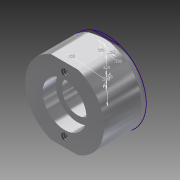
# Autodesk Inventor part: Pnuematic Connector
Saved by Autodesk Inventor 2013 (Build 170138000, 138)
## iProperties
Created: 2013-06-07
Part Number: Pnuematic Connector
Material: Generic
Document SubType Name: Modeling
Designer: mvarma
Density: 1 g/cm^3
Author: mvarma
Autodesk Inventor part; units mm, degrees
ref_plane "YZ Plane" through (0, 0, 0) normal (1, 0, 0) x (0, 1, 0)
ref_plane "XZ Plane" through (0, 0, 0) normal (0, 1, 0) x (-1, 0, 0)
ref_plane "XY Plane" through (0, 0, 0) normal (0, 0, 1) x (1, 0, 0)
sketch "Sketch1" plane through (0, 0, 0) normal (0, 0, 1) x (1, 0, 0)
  circle A0 centre (0, 0) radius 3.175
  line L0 (-1.508, 2.794) -> (1.508, 2.794)
  line L1 (-3.175, 0) -> (0, 0)
  line L2 (0, 0) -> (3.175, 0)
  line L3 (-1.508, -2.794) -> (1.508, -2.794)
  circle A1 centre (0, 0) radius 7.9375
  arc A2 (-4.892, 13.4239) -> (-4.892, -13.4239) centre (0, 0) ccw
  circle A3 centre (0, 10.0965) radius 1.905 construction
  circle A4 centre (0, 10.0965) radius 3.3274 construction
  circle A5 centre (0, 0) radius 10.0965 construction
  line L4 (0, 0) -> (0, 10.0965) construction
  line L5 (0, -10.0965) -> (0, 0) construction
  line L6 (-4.892, 13.4239) -> (4.892, 13.4239)
  arc A6 (4.892, 13.4239) -> (-4.892, 13.4239) centre (0, 0) ccw
  circle A7 centre (0, -10.0965) radius 3.3274 construction
  line L7 (-4.892, -13.4239) -> (4.892, -13.4239)
  arc A8 (4.892, -13.4239) -> (4.892, 13.4239) centre (0, 0) ccw
  arc A9 (-4.892, -13.4239) -> (4.892, -13.4239) centre (0, 0) ccw
  dimension "d0" = 6.35
  dimension "d1" = 5.588
  dimension "d2" = 15.875
  dimension "d4" = 3.81
  dimension "d5" = 6.6548
  dimension "d7" = 2.159
  dimension "d8" = 14.2875
  constraints: 17 point on circle, 16 end point, 10 centre point, 8 coincident, 2 collinear, 2 parallel, 2 tangent, 1 equal radius, 1 horizontal, 1 perpendicular, 1 vertical, 1 other
  measures "d0" diameter of A0
  measures "d1" distance between parallel lines of L3 L0
  measures "d2" diameter of A1
  measures "d4" diameter of A3
  measures "d5" diameter of A4
  measures "d7" radial gap between concentric circles of A1 A5
  measures "d8" radius of A2
extrude "Extrusion1" add sketch "Sketch1" along normal blind 15.2781 and the other way blind 3.175 contours L6 A8 L7 A2 | A6 L6 | L7 A9
extrude "Extrusion2" add sketch "Sketch1" against normal blind 3.175 contours L0 A0 | A0 L3 | A1
extrude "Extrusion3" add sketch "Sketch1" along normal blind 3.175 contours L2 L1 A0 L0 | A0 L3 L1 L2 | L0 A0 | A0 L3 | A1
hole "Hole1" at (0, 0, 0) direction (0, 0, 1) diameter 3.302 end through all thread size "8-32 UNC" class "2B" standard "ANSI Unified Screw Threads"
sketch "Sketch2" plane through (0, 0, 3.175) normal (0, 0, 1) x (1, 0, 0)
  circle A0 centre (0, 0) radius 7.9375 projected
  circle A1 centre (0, 0) radius 3.429 construction
  circle A2 centre (0, 0) radius 5.715
  dimension "d22" = 6.858
  dimension "d23" = 11.43
  constraints: 2 centre point, 2 coincident
  measures "d22" diameter of A1
  measures "d23" diameter of A2
extrude "Extrusion4" add sketch "Sketch2" along normal blind 7.3406
sketch "Sketch3" plane through (0, 0, 15.2781) normal (0, 0, 1) x (1, 0, 0)
  point P0 (0, -10.0965)
  point P1 (0, 10.0965)
hole "Hole2" at (0, 10.0965, 15.2781) at (0, -10.0965, 15.2781) direction (0, 0, -1) diameter 2.6416 depth 9.525 tip angle 118 thread size "6-32 UNC" class "2B" standard "ANSI Unified Screw Threads"
chamfer "Chamfer1" distance 4.7625 angle 45 1 edges at (-4.892, 13.4239, -3.175)
extrude "Extrusion5" cut sketch "Sketch1" along normal up to surface (15.2781 mm away) contours A6 L6 | L7 A9
body "Solid1"
